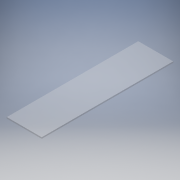
# Autodesk Inventor part: AccessFloor2
Saved by Autodesk Inventor 2018 (Build 220112000, 112)
## iProperties
Created: 2013-02-21
Part Number: AccessFloor2
Material: PVC-U
Document SubType Name: Modeling
Designer: Neef
Mass: 592.561 g
Surface Area: 1495.34 cm^2
Volume: 423.258 cm^3
Density: 1.29 g/cm^3
Appearance: Smooth - White
Author: Neef
Autodesk Inventor part; units mm, degrees
ref_plane "YZ Plane" through (0, 0, 0) normal (1, 0, 0) x (0, 1, 0)
ref_plane "XZ Plane" through (0, 0, 0) normal (0, 1, 0) x (-1, 0, 0)
ref_plane "XY Plane" through (0, 0, 0) normal (0, 0, 1) x (1, 0, 0)
sketch "Skizze1" plane through (0, 0, 0) normal (0, 0, 1) x (1, 0, 0)
  line L0 (0, 408.1) -> (0, -408.1) projected
  line L1 (-108.5, 0) -> (108.5, 0) projected
  line L2 (-77.5, -291.5) -> (77.5, -291.5)
  line L3 (77.5, -291.5) -> (77.5, 291.5)
  line L4 (77.5, 291.5) -> (-77.5, 291.5)
  line L5 (-77.5, 291.5) -> (-77.5, -291.5)
  point P0 (0, 0)
  point P1 (0, -291.5)
  point P2 (-77.5, 0)
  dimension "d0" = 583
  dimension "d1" = 155
  constraints: 8 end point, 2 midpoint, 2 parallel, 2 point on line, 1 horizontal, 1 perpendicular
  measures "d0" distance of L4.end L2.start
  measures "d1" distance of L2.start L2.end
extrude "Extrusion1" add sketch "Skizze1" along normal blind 6
